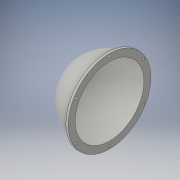
# Autodesk Inventor part: ROV Dome 4''
Saved by Autodesk Inventor 2016 (Build 200138000, 138)
## iProperties
Created: 2017-02-01
Part Number: ROV Dome 4''
Material: Generic
Document SubType Name: Modeling
Designer: Student
Density: 1 g/cm^3
Appearance: Default
Mass: 45.4784 g
Surface Area: 368.897 cm^2
Volume: 45.4784 cm^3
Author: Student
Autodesk Inventor part; units mm, degrees
ref_plane "YZ Plane" through (0, 0, 0) normal (1, 0, 0) x (0, 1, 0)
ref_plane "XZ Plane" through (0, 0, 0) normal (0, 1, 0) x (-1, 0, 0)
ref_plane "XY Plane" through (0, 0, 0) normal (0, 0, 1) x (1, 0, 0)
sketch "Sketch1" plane through (0, 0, 0) normal (0, 1, 0) x (-1, 0, 0)
  arc A0 (50.8, 0) -> (0, 50.8) centre (0, 0) ccw
  line L0 (0, 50.8) -> (0, 57.15)
  line L1 (-3.175, 57.15) -> (-3.175, 47.519)
  arc A1 (47.625, 0) -> (-3.175, 47.519) centre (0, 0) ccw
  line L2 (0, 57.15) -> (-3.175, 57.15)
  line L3 (50.8, 0) -> (47.6207, 0)
  line L4 (-3.175, 47.519) -> (-3.175, -38.7151)
  line L5 (50.8, 0) -> (-3.175, 0) construction
  dimension "d0" = 50.8
  dimension "d5" = 3.175
  dimension "d19" = 57.15
  dimension "d20" = 3.175
  dimension "d21" = 6.35
  constraints: 12 end point, 4 point on circle, 2 centre point, 2 horizontal, 2 point on line, 2 vertical, 1 coincident, 1 perpendicular
  measures "d0" distance of point (0, 0) L0.start
  measures "d5" radial gap between concentric circles of A0 A1
  measures "d19" vertical distance of point (0, 0) L1.start
  measures "d20" distance between parallel lines of L1 L0
  measures "d21" distance of L0.start L0.end
revolve "Revolution1" add sketch "Sketch1" angle 360 about axis through (-50.8, 0, 0) along (1, 0, 0)
sketch "Sketch2" plane through (0, 0, 0) normal (-1, 0, 0) x (0, 0, 1)
  circle A0 centre (0, 53.975) radius 1.7526
  circle A1 centre (0, 0) radius 50.8 projected
  circle A2 centre (-46.7437, 26.9875) radius 1.7526
  circle A3 centre (-46.7437, -26.9875) radius 1.7526
  circle A4 centre (0, -53.975) radius 1.7526
  circle A5 centre (46.7437, -26.9875) radius 1.7526
  circle A6 centre (46.7437, 26.9875) radius 1.7526
  point P0 (0, 0)
  dimension "d10" = 3.5052
  dimension "d12" = 53.975
  dimension "d15" = 360
  constraints: 6 centre point, 13 other
  measures "d10" diameter of A0
  measures "d12" distance of point (0, 0) A0.centre
extrude "Extrusion1" cut sketch "Sketch2" against normal blind 254 contours A0 | A2 | A3 | A4 | A5 | A6
body "Solid1"
